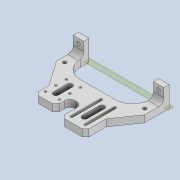
# Autodesk Inventor part: cpr_shell_2
Saved by Autodesk Inventor 2020 (Build 240168000, 168)
## iProperties
Created: 2021-10-08
Part Number: cpr_shell_2
Material: Generic
Document SubType Name: Modeling
Designer: Shuang Peng
Density: 1 g/cm^3
Appearance: Default
Author: Shuang Peng
Autodesk Inventor part; units mm, degrees
ref_plane "YZ Plane" through (0, 0, 0) normal (1, 0, 0) x (0, 1, 0)
ref_plane "XZ Plane" through (0, 0, 0) normal (0, 1, 0) x (-1, 0, 0)
ref_plane "XY Plane" through (0, 0, 0) normal (0, 0, 1) x (1, 0, 0)
sketch "Sketch1" plane through (0, 0, 0) normal (0, 0, 1) x (1, 0, 0)
  circle A0 centre (23, -7.5) radius 1 projected
  circle A1 centre (23, 7.5) radius 1 projected
  line L0 (6, -13) -> (6, -16) projected
  line L1 (6, -16) -> (26, -16) projected
  line L2 (26, -16) -> (26, 16) projected
  line L3 (26, 16) -> (6, 16) projected
  line L4 (6, 16) -> (6, 13) projected
  line L5 (6, 13) -> (20, 13) projected
  line L6 (20, 13) -> (20, -13) projected
  line L7 (20, -13) -> (6, -13) projected
  circle A2 centre (-23, -7.5) radius 1 projected
  circle A3 centre (-23, 7.5) radius 1 projected
  line L8 (-6, -16) -> (-6, -13) projected
  line L9 (-6, -13) -> (-20, -13) projected
  line L10 (-20, -13) -> (-20, 13) projected
  line L11 (-20, 13) -> (-6, 13) projected
  line L12 (-6, 13) -> (-6, 16) projected
  line L13 (-6, 16) -> (-26, 16) projected
  line L14 (-26, 16) -> (-26, -16) projected
  line L15 (-26, -16) -> (-6, -16) projected
  line L16 (23, 7.5) -> (23, -7.5)
  line L17 (26, -10) -> (20, -10)
  line L18 (20, -10) -> (20, 10)
  line L19 (20, 10) -> (26, 10)
  line L20 (26, 10) -> (26, -10)
  line L21 (26, -10) -> (20, 10) construction
  line L22 (20, -10) -> (26, 10) construction
  line L23 (-23, 7.5) -> (-23, -7.5)
  line L24 (-20, -10) -> (-26, -10)
  line L25 (-26, -10) -> (-26, 10)
  line L26 (-26, 10) -> (-20, 10)
  line L27 (-20, 10) -> (-20, -10)
  line L28 (-20, -10) -> (-26, 10) construction
  line L29 (-26, -10) -> (-20, 10) construction
  point P0 (0, 0)
  point P1 (23, 0)
  point P2 (-23, 0)
  point P3 (-26, 10)
  dimension "d0" = 6
  dimension "d1" = 20
  dimension "d2" = 6
  dimension "d3" = 20
  constraints: 28 end point, 6 midpoint, 5 parallel, 4 perpendicular, 1 vertical
  measures "d0" distance of L17.start L17.end
  measures "d1" distance of L17.end L18.end
  measures "d2" distance of L24.start L24.end
  measures "d3" distance of L24.end L25.end
extrude "Extrusion1" add sketch "Sketch1" along normal blind 3 contours L6 L19 L2 L17 | L14 L26 L10 L24
ref_plane "Work Plane1" through (20, 0, 0) normal (0, -1, 0) x (1, 0, 0)
sketch "Sketch2" plane through (20, 0, 0) normal (0, -1, 0) x (1, 0, 0)
  line L0 (0, 0) -> (6, 0) projected
  line L1 (6, 0) -> (6, 3) projected
  line L2 (0, 3) -> (6, 3) projected
  line L3 (0, 0) -> (0, 3) projected
  line L4 (-46, 0) -> (-40, 0) projected
  line L5 (-40, 0) -> (-40, 3) projected
  line L6 (-46, 3) -> (-40, 3) projected
  line L7 (-46, 0) -> (-46, 3) projected
  line L8 (-40, 0) -> (-40, 3) projected
  line L9 (-40, 3) -> (0, 3)
  line L10 (0, 3) -> (0, 15)
  line L11 (0, 15) -> (-40, 15)
  line L12 (-40, 15) -> (-40, 3)
  line L13 (0, 3) -> (6, 3) projected
  line L14 (6, 3) -> (-46, 3)
  line L15 (-46, 3) -> (-46, 27)
  line L16 (-46, 27) -> (6, 27)
  line L17 (6, 27) -> (6, 3)
  point P0 (-20, 0)
  dimension "d6" = 40
  dimension "d7" = 12
  dimension "d8" = 52
  dimension "d9" = 24
  constraints: 16 end point, 4 parallel, 2 horizontal, 2 perpendicular
  measures "d6" distance of L11.end L10.end
  measures "d7" distance of L10.end L9.end
  measures "d8" distance of L15.end L16.end
  measures "d9" distance of L14.end L15.end
extrude "Extrusion2" add sketch "Sketch2" along normal mid plane 4 contours L10 L11 L12 L6 L15 L16 L17 L2
sketch "Sketch3" plane through (20, -2, 0) normal (0, -1, 0) x (1, 0, 0)
  line L0 (-30, 11) -> (-30, 39)
  line L1 (-40, 3) -> (-40, 15) projected
  line L2 (-40, 15) -> (0, 15) projected
  line L3 (0, 15) -> (0, 3) projected
  line L4 (6, 3) -> (0, 3) projected
  line L5 (6, 3) -> (6, 27) projected
  line L6 (6, 27) -> (-46, 27) projected
  line L7 (-46, 27) -> (-46, 3) projected
  line L8 (-40, 3) -> (-46, 3) projected
  line L9 (-36, 39) -> (-24, 39)
  line L10 (-24, 39) -> (-24, 15)
  line L11 (-24, 15) -> (-36, 15)
  line L12 (-36, 15) -> (-36, 39)
  line L13 (-46, 27) -> (6, 27) projected
  line L14 (-36, 39) -> (-24, 15) construction
  line L15 (-24, 39) -> (-36, 15) construction
  line L16 (6, 27) -> (-46, 27) projected
  line L17 (-10, 39) -> (-10, 11)
  line L18 (-16, 39) -> (-4, 39)
  line L19 (-4, 39) -> (-4, 15)
  line L20 (-4, 15) -> (-16, 15)
  line L21 (-16, 15) -> (-16, 39)
  line L22 (-16, 39) -> (-4, 15) construction
  line L23 (-4, 39) -> (-16, 15) construction
  point P0 (-20, 0)
  point P1 (-30, 27)
  point P2 (-10, 27)
  point P3 (-16, 27)
  point P4 (-4, 27)
  point P5 (-24, 27)
  point P6 (-36, 27)
  dimension "d12" = 12
  dimension "d13" = 24
  dimension "d14" = 12
  dimension "d15" = 24
  constraints: 28 end point, 4 midpoint, 4 parallel, 4 perpendicular, 4 point on line, 2 vertical, 4 other
  measures "d12" distance of L9.start L9.end
  measures "d13" distance of L9.end L10.end
  measures "d14" distance of L18.start L18.end
  measures "d15" distance of L18.end L19.end
extrude "Extrusion3" add sketch "Sketch3" against normal up to surface (4 mm away) contours L6 L12 L9 L0 | L0 L9 L10 L6 | L21 L18 L17 L6 | L17 L18 L19 L6
sketch "Sketch4" plane through (20, -2, 0) normal (0, -1, 0) x (1, 0, 0)
  line L0 (-40, 3) -> (-40, 15) projected
  line L1 (-40, 15) -> (0, 15) projected
  line L2 (0, 15) -> (0, 3) projected
  line L3 (6, 3) -> (0, 3) projected
  line L4 (6, 3) -> (6, 27) projected
  line L5 (6, 27) -> (-4, 27) projected
  line L6 (-4, 27) -> (-4, 39) projected
  line L7 (-4, 39) -> (-16, 39) projected
  line L8 (-16, 39) -> (-16, 27) projected
  line L9 (-16, 27) -> (-24, 27) projected
  line L10 (-24, 27) -> (-24, 39) projected
  line L11 (-24, 39) -> (-36, 39) projected
  line L12 (-36, 39) -> (-36, 27) projected
  line L13 (-36, 27) -> (-46, 27) projected
  line L14 (-46, 27) -> (-46, 3) projected
  line L15 (-40, 3) -> (-46, 3) projected
  line L16 (-46, 0) -> (-40, 0) projected
  line L17 (-40, 0) -> (-40, 3) projected
  line L18 (-46, 3) -> (-40, 3) projected
  line L19 (-46, 0) -> (-46, 3) projected
  line L20 (0, 0) -> (6, 0) projected
  line L21 (6, 0) -> (6, 3) projected
  line L22 (0, 3) -> (6, 3) projected
  line L23 (0, 0) -> (0, 3) projected
  point P0 (-20, 0)
extrude "Extrusion4" cut sketch "Sketch4" along normal blind 12 contours L17 L16 L19 L15 | L3 L21 L20 L23
thicken "Thicken1" operation add thickness 4 both sides no extend neighbours yes toward (0, 0, -1) faces at (-8, -0.6667, 39)
sketch "Sketch5" plane through (20, 2, 0) normal (0, 1, 0) x (1, 0, 0)
  circle A0 centre (-6, -31) radius 0.6 projected
  circle A1 centre (-6, -25) radius 0.6 projected
  circle A2 centre (-6, -19) radius 0.6 projected
  circle A3 centre (-14, -31) radius 0.6 projected
  circle A4 centre (-14, -25) radius 0.6 projected
  circle A5 centre (-14, -19) radius 0.6 projected
  line L0 (-6, -19) -> (-6, -36) construction
  line L1 (-6.65, -19) -> (-6.65, -36)
  line L2 (-5.35, -36) -> (-5.35, -19)
  arc A6 (-5.35, -19) -> (-6.65, -19) centre (-6, -19) ccw
  arc A7 (-6.65, -36) -> (-5.35, -36) centre (-6, -36) ccw
  line L3 (-14, -19) -> (-14, -36) construction
  line L4 (-14.65, -19) -> (-14.65, -36)
  line L5 (-13.35, -36) -> (-13.35, -19)
  arc A8 (-13.35, -19) -> (-14.65, -19) centre (-14, -19) ccw
  arc A9 (-14.65, -36) -> (-13.35, -36) centre (-14, -36) ccw
  point P0 (-20, 0)
  point P1 (-6, -27.5)
  point P2 (-14, -27.5)
  dimension "d22" = 17
  dimension "d23" = 1.3
  dimension "d24" = 17
  dimension "d25" = 1.3
  constraints: 16 end point, 8 point on circle, 8 tangent, 4 centre point, 2 midpoint, 2 parallel, 2 vertical
  measures "d22" distance of L0.start L0.end
  measures "d23" diameter of A7
  measures "d24" distance of L3.start L3.end
  measures "d25" diameter of A9
extrude "Extrusion5" cut sketch "Sketch5" against normal blind 12 contours A0 | A1 | A2 | A3 | A4 | A5 | A6 L2 A7 L1 | A8 L5 A9 L4
sketch "Sketch6" plane through (20, 2, 0) normal (0, 1, 0) x (1, 0, 0)
  line L0 (-14.65, -36) -> (-14.65, -19) projected
  arc A0 (-13.35, -19) -> (-14.65, -19) centre (-14, -19) ccw projected
  line L1 (-13.35, -19) -> (-13.35, -36) projected
  arc A1 (-14.65, -36) -> (-13.35, -36) centre (-14, -36) ccw projected
  arc A2 (-5.35, -19) -> (-6.65, -19) centre (-6, -19) ccw projected
  line L2 (-5.35, -19) -> (-5.35, -36) projected
  arc A3 (-6.65, -36) -> (-5.35, -36) centre (-6, -36) ccw projected
  line L3 (-6.65, -36) -> (-6.65, -19) projected
  line L4 (-40, -15) -> (-40, -3) projected
  line L5 (-46, -3) -> (-40, -3) projected
  line L6 (-46, -3) -> (-46, -27) projected
  line L7 (-46, -27) -> (-36, -27) projected
  line L8 (-36, -35) -> (-36, -27) projected
  line L9 (-24, -35) -> (-36, -35) projected
  line L10 (-24, -27) -> (-24, -35) projected
  line L11 (-24, -27) -> (-16, -27) projected
  line L12 (-16, -39) -> (-16, -27) projected
  line L13 (-4, -39) -> (-16, -39) projected
  line L14 (-4, -27) -> (-4, -39) projected
  line L15 (-4, -27) -> (6, -27) projected
  line L16 (6, -27) -> (6, -3) projected
  line L17 (0, -3) -> (6, -3) projected
  line L18 (0, -3) -> (0, -15) projected
  line L19 (0, -15) -> (-40, -15) projected
  line L20 (-26, -15) -> (-25, -16) projected
  line L21 (-28.0404, -15) -> (-26, -15) projected
  line L22 (-28.0404, -35) -> (-28.0404, -15) projected
  line L23 (-26, -35) -> (-28.0404, -35) projected
  line L24 (-25, -34) -> (-26, -35) projected
  line L25 (-25, -33) -> (-25, -34) projected
  arc A4 (-24.5, -32.5) -> (-25, -33) centre (-24.5, -33) ccw projected
  line L26 (-24.5, -32.5) -> (-24, -32.5) projected
  line L27 (-24, -32.5) -> (-24, -29.5) projected
  line L28 (-24, -29.5) -> (-24.5, -29.5) projected
  arc A5 (-25, -29) -> (-24.5, -29.5) centre (-24.5, -29) ccw projected
  line L29 (-25, -27) -> (-25, -29) projected
  arc A6 (-24.5, -26.5) -> (-25, -27) centre (-24.5, -27) ccw projected
  line L30 (-24.5, -26.5) -> (-24, -26.5) projected
  line L31 (-24, -26.5) -> (-24, -23.5) projected
  line L32 (-24, -23.5) -> (-24.5, -23.5) projected
  arc A7 (-25, -23) -> (-24.5, -23.5) centre (-24.5, -23) ccw projected
  line L33 (-25, -21) -> (-25, -23) projected
  arc A8 (-24.5, -20.5) -> (-25, -21) centre (-24.5, -21) ccw projected
  line L34 (-24.5, -20.5) -> (-24, -20.5) projected
  line L35 (-24, -20.5) -> (-24, -17.5) projected
  line L36 (-24, -17.5) -> (-24.5, -17.5) projected
  arc A9 (-25, -17) -> (-24.5, -17.5) centre (-24.5, -17) ccw projected
  line L37 (-25, -16) -> (-25, -17) projected
  circle A10 centre (-26, -19) radius 0.6 projected
  circle A11 centre (-26, -25) radius 0.6 projected
  circle A12 centre (-26, -31) radius 0.6 projected
  line L38 (-35, -16) -> (-34, -15) projected
  line L39 (-35, -16) -> (-35, -17) projected
  arc A13 (-35.5, -17.5) -> (-35, -17) centre (-35.5, -17) ccw projected
  line L40 (-36, -17.5) -> (-35.5, -17.5) projected
  line L41 (-36, -20.5) -> (-36, -17.5) projected
  line L42 (-35.5, -20.5) -> (-36, -20.5) projected
  arc A14 (-35, -21) -> (-35.5, -20.5) centre (-35.5, -21) ccw projected
  line L43 (-35, -21) -> (-35, -23) projected
  arc A15 (-35.5, -23.5) -> (-35, -23) centre (-35.5, -23) ccw projected
  line L44 (-36, -23.5) -> (-35.5, -23.5) projected
  line L45 (-36, -26.5) -> (-36, -23.5) projected
  line L46 (-35.5, -26.5) -> (-36, -26.5) projected
  arc A16 (-35, -27) -> (-35.5, -26.5) centre (-35.5, -27) ccw projected
  line L47 (-35, -27) -> (-35, -29) projected
  arc A17 (-35.5, -29.5) -> (-35, -29) centre (-35.5, -29) ccw projected
  line L48 (-36, -29.5) -> (-35.5, -29.5) projected
  line L49 (-36, -32.5) -> (-36, -29.5) projected
  line L50 (-35.5, -32.5) -> (-36, -32.5) projected
  arc A18 (-35, -33) -> (-35.5, -32.5) centre (-35.5, -33) ccw projected
  line L51 (-35, -33) -> (-35, -34) projected
  line L52 (-34, -35) -> (-35, -34) projected
  line L53 (-31.9596, -35) -> (-34, -35) projected
  line L54 (-31.9596, -15) -> (-31.9596, -35) projected
  line L55 (-34, -15) -> (-31.9596, -15) projected
  circle A19 centre (-34, -19) radius 0.6 projected
  circle A20 centre (-34, -25) radius 0.6 projected
  circle A21 centre (-34, -31) radius 0.6 projected
  point P0 (-20, 0)
extrude "Extrusion6" cut sketch "Sketch6" against normal blind 12 contours A10 | A11 | A12 | A19 | A20 | A21
thicken "Thicken2" operation add thickness 1 both sides no extend neighbours yes toward (1, 0, 0) faces at (16, -0.6667, 31)
thicken "Thicken3" operation add thickness 1 both sides no extend neighbours yes toward (-1, 0, 0) faces at (4, -0.6667, 35)
fillet "Fillet1" radius 10 2 edges at (-20, 0, 15) (20, 0, 15)
sketch "Sketch7" plane through (20, 2, 0) normal (0, 1, 0) x (1, 0, 0)
  circle A0 centre (-26, -19) radius 0.6 projected
  circle A1 centre (-34, -19) radius 0.6 projected
  circle A2 centre (-26, -25) radius 0.6 projected
  circle A3 centre (-34, -31) radius 0.6 projected
  circle A4 centre (-34, -25) radius 0.6 projected
  circle A5 centre (-26, -31) radius 0.6 projected
  line L0 (-14.65, -36) -> (-14.65, -19) projected
  arc A6 (-13.35, -19) -> (-14.65, -19) centre (-14, -19) ccw projected
  line L1 (-13.35, -19) -> (-13.35, -36) projected
  arc A7 (-14.65, -36) -> (-13.35, -36) centre (-14, -36) ccw projected
  arc A8 (-6.65, -36) -> (-5.35, -36) centre (-6, -36) ccw projected
  line L2 (-6.65, -36) -> (-6.65, -19) projected
  arc A9 (-5.35, -19) -> (-6.65, -19) centre (-6, -19) ccw projected
  line L3 (-5.35, -19) -> (-5.35, -36) projected
  line L4 (-40, -5) -> (-40, -3) projected
  line L5 (-46, -3) -> (-40, -3) projected
  line L6 (-46, -3) -> (-46, -27) projected
  line L7 (-46, -27) -> (-36, -27) projected
  line L8 (-36, -35) -> (-36, -27) projected
  line L9 (-24, -35) -> (-36, -35) projected
  line L10 (-24, -27) -> (-24, -35) projected
  line L11 (-24, -27) -> (-17, -27) projected
  line L12 (-17, -39) -> (-17, -27) projected
  line L13 (-3, -39) -> (-17, -39) projected
  line L14 (-3, -27) -> (-3, -39) projected
  line L15 (-3, -27) -> (6, -27) projected
  line L16 (6, -27) -> (6, -3) projected
  line L17 (0, -3) -> (6, -3) projected
  line L18 (0, -3) -> (0, -5) projected
  arc A10 (-10, -15) -> (0, -5) centre (-10, -5) ccw projected
  line L19 (-10, -15) -> (-30, -15) projected
  arc A11 (-40, -5) -> (-30, -15) centre (-30, -5) ccw projected
  line L20 (-36, -35) -> (-36, -27) projected
  line L21 (-36, -27) -> (-46, -12.7185)
  line L22 (-46, 0) -> (-46, -27) projected
  line L23 (-3, -27) -> (6, -14.1467)
  point P0 (-20, 0)
  dimension "d35" = 55
  dimension "d36" = 55
  constraints: 4 end point, 2 point on line
  measures "d35" angle of L7 L21
  measures "d36" angle of L15 L23
extrude "Extrusion7" cut sketch "Sketch7" against normal blind 12 contours L21 L7 L6 | L16 L15 L23
fillet "Fillet2" radius 3 2 edges at (-23, 2, 3) (23, 2, 3)
chamfer "Chamfer1" distance 2 angle 45 4 edges at (-16, 0, 35) (-4, 0, 35) (3, 0, 39) (17, 0, 39)
fillet "Fillet3" radius 3 2 edges at (-4, 0, 27) (3, 0, 27)
sketch "Sketch8" plane through (20, 2, 0) normal (0, 1, 0) x (1, 0, 0)
  line L0 (-3, -37) -> (-5, -39) projected
  line L1 (-3, -27) -> (-3, -37) projected
  line L2 (-3, -27) -> (6, -14.1467) projected
  line L3 (6, -14.1467) -> (6, -6) projected
  line L4 (-0.0501, -6) -> (6, -6) projected
  arc A0 (-10, -15) -> (-0.0501, -6) centre (-10, -5) ccw projected
  line L5 (-10, -15) -> (-30, -15) projected
  arc A1 (-39.9499, -6) -> (-30, -15) centre (-30, -5) ccw projected
  line L6 (-46, -6) -> (-39.9499, -6) projected
  line L7 (-46, -6) -> (-46, -12.7185) projected
  line L8 (-46, -12.7185) -> (-36, -27) projected
  line L9 (-36, -33) -> (-36, -27) projected
  line L10 (-34, -35) -> (-36, -33) projected
  line L11 (-26, -35) -> (-34, -35) projected
  line L12 (-24, -33) -> (-26, -35) projected
  line L13 (-24, -30) -> (-24, -33) projected
  arc A2 (-21, -27) -> (-24, -30) centre (-21, -30) ccw projected
  line L14 (-21, -27) -> (-20, -27) projected
  arc A3 (-17, -30) -> (-20, -27) centre (-20, -30) ccw projected
  line L15 (-17, -37) -> (-17, -30) projected
  line L16 (-15, -39) -> (-17, -37) projected
  line L17 (-5, -39) -> (-15, -39) projected
  circle A4 centre (-26, -19) radius 0.6 projected
  circle A5 centre (-34, -19) radius 0.6 projected
  circle A6 centre (-26, -25) radius 0.6 projected
  circle A7 centre (-34, -31) radius 0.6 projected
  circle A8 centre (-34, -25) radius 0.6 projected
  circle A9 centre (-26, -31) radius 0.6 projected
  line L18 (-14.65, -36) -> (-14.65, -19) projected
  arc A10 (-13.35, -19) -> (-14.65, -19) centre (-14, -19) ccw projected
  line L19 (-13.35, -19) -> (-13.35, -36) projected
  arc A11 (-14.65, -36) -> (-13.35, -36) centre (-14, -36) ccw projected
  arc A12 (-6.65, -36) -> (-5.35, -36) centre (-6, -36) ccw projected
  line L20 (-6.65, -36) -> (-6.65, -19) projected
  arc A13 (-5.35, -19) -> (-6.65, -19) centre (-6, -19) ccw projected
  line L21 (-5.35, -19) -> (-5.35, -36) projected
  circle A14 centre (-34, -31) radius 0.6 projected
  circle A15 centre (-26, -19) radius 0.6 projected
  line L22 (-34, -31) -> (-26, -19)
  circle A16 centre (-26, -31) radius 0.6 projected
  line L23 (-26, -31) -> (-34, -19)
  line L24 (-30, -29) -> (-30, -21) construction
  line L25 (-28.5, -29) -> (-28.5, -21)
  line L26 (-31.5, -21) -> (-31.5, -29)
  arc A17 (-31.5, -29) -> (-28.5, -29) centre (-30, -29) ccw
  arc A18 (-28.5, -21) -> (-31.5, -21) centre (-30, -21) ccw
  arc A19 (-5.35, -19) -> (-6.65, -19) centre (-6, -19) ccw projected
  line L27 (-14, -36) -> (-6, -19)
  arc A20 (-13.35, -19) -> (-14.65, -19) centre (-14, -19) ccw projected
  line L28 (-6, -19) -> (-14, -19)
  arc A21 (-6.65, -36) -> (-5.35, -36) centre (-6, -36) ccw projected
  line L29 (-14, -19) -> (-6, -36)
  line L30 (-10, -32.5) -> (-10, -22.5) construction
  line L31 (-8.5, -32.5) -> (-8.5, -22.5)
  line L32 (-11.5, -22.5) -> (-11.5, -32.5)
  arc A22 (-11.5, -32.5) -> (-8.5, -32.5) centre (-10, -32.5) ccw
  arc A23 (-8.5, -22.5) -> (-11.5, -22.5) centre (-10, -22.5) ccw
  point P0 (-20, 0)
  point P1 (-30, -25)
  point P2 (-10, -27.5)
  dimension "d44" = 4
  dimension "d45" = 3
  dimension "d46" = 5
  dimension "d47" = 3
  constraints: 26 end point, 8 point on circle, 8 tangent, 4 centre point, 4 midpoint, 2 parallel, 2 vertical, 1 horizontal
  measures "d44" distance of point (-30, -25) L24.end
  measures "d45" diameter of A18
  measures "d46" distance of point (-10, -27.5) L30.end
  measures "d47" diameter of A23
extrude "Extrusion8" cut sketch "Sketch8" against normal blind 12 contours L32 L29 L27 | L27 L29 L31 A22 L32 | L32 A23 L31 L27 L29 | L27 L31 L29 | L26 L23 L22 | L22 L23 L25 A17 L26 | L23 L26 A18 L25 L22 | L22 L25 L23
sketch "Sketch9" plane through (20, 2, 0) normal (0, 1, 0) x (1, 0, 0)
  line L0 (-11.5, -32.5) -> (-11.5, -22.5) projected
  arc A0 (-8.5, -22.5) -> (-11.5, -22.5) centre (-10, -22.5) ccw projected
  line L1 (-8.5, -22.5) -> (-8.5, -32.5) projected
  arc A1 (-11.5, -32.5) -> (-8.5, -32.5) centre (-10, -32.5) ccw projected
  line L2 (-31.5, -29) -> (-31.5, -21) projected
  arc A2 (-28.5, -21) -> (-31.5, -21) centre (-30, -21) ccw projected
  line L3 (-28.5, -21) -> (-28.5, -29) projected
  arc A3 (-31.5, -29) -> (-28.5, -29) centre (-30, -29) ccw projected
  line L4 (-3, -37) -> (-5, -39) projected
  line L5 (-3, -27) -> (-3, -37) projected
  line L6 (-3, -27) -> (6, -14.1467) projected
  line L7 (6, -14.1467) -> (6, -6) projected
  line L8 (-0.0501, -6) -> (6, -6) projected
  arc A4 (-10, -15) -> (-0.0501, -6) centre (-10, -5) ccw projected
  line L9 (-10, -15) -> (-30, -15) projected
  arc A5 (-39.9499, -6) -> (-30, -15) centre (-30, -5) ccw projected
  line L10 (-46, -6) -> (-39.9499, -6) projected
  line L11 (-46, -6) -> (-46, -12.7185) projected
  line L12 (-46, -12.7185) -> (-36, -27) projected
  line L13 (-36, -33) -> (-36, -27) projected
  line L14 (-34, -35) -> (-36, -33) projected
  line L15 (-26, -35) -> (-34, -35) projected
  line L16 (-24, -33) -> (-26, -35) projected
  line L17 (-24, -30) -> (-24, -33) projected
  arc A6 (-21, -27) -> (-24, -30) centre (-21, -30) ccw projected
  line L18 (-21, -27) -> (-20, -27) projected
  arc A7 (-17, -30) -> (-20, -27) centre (-20, -30) ccw projected
  line L19 (-17, -37) -> (-17, -30) projected
  line L20 (-15, -39) -> (-17, -37) projected
  line L21 (-5, -39) -> (-15, -39) projected
  circle A8 centre (-26, -19) radius 0.6 projected
  circle A9 centre (-34, -19) radius 0.6 projected
  circle A10 centre (-26, -25) radius 0.6 projected
  circle A11 centre (-34, -31) radius 0.6 projected
  circle A12 centre (-34, -25) radius 0.6 projected
  circle A13 centre (-26, -31) radius 0.6 projected
  line L22 (-14.65, -36) -> (-14.65, -19) projected
  arc A14 (-13.35, -19) -> (-14.65, -19) centre (-14, -19) ccw projected
  line L23 (-13.35, -19) -> (-13.35, -36) projected
  arc A15 (-14.65, -36) -> (-13.35, -36) centre (-14, -36) ccw projected
  arc A16 (-6.65, -36) -> (-5.35, -36) centre (-6, -36) ccw projected
  line L24 (-6.65, -36) -> (-6.65, -19) projected
  arc A17 (-5.35, -19) -> (-6.65, -19) centre (-6, -19) ccw projected
  line L25 (-5.35, -19) -> (-5.35, -36) projected
  line L26 (-0.0501, -6) -> (6, -6) projected
  line L27 (2.9749, -6) -> (2.9749, -11)
  circle A18 centre (2.9749, -11) radius 1
  line L28 (-46, -6) -> (-39.9499, -6) projected
  line L29 (-42.9749, -6) -> (-42.9749, -11)
  circle A19 centre (-42.9749, -11) radius 1
  point P0 (-20, 0)
  dimension "d50" = 5
  dimension "d51" = 2
  dimension "d52" = 5
  dimension "d53" = 2
  constraints: 4 end point, 2 centre point, 2 coincident, 2 midpoint, 2 vertical
  measures "d50" distance of L27.start L27.end
  measures "d51" diameter of A18
  measures "d52" distance of L29.start L29.end
  measures "d53" diameter of A19
extrude "Extrusion9" cut sketch "Sketch9" against normal blind 12 contours A18 | A19
body "Solid1"
